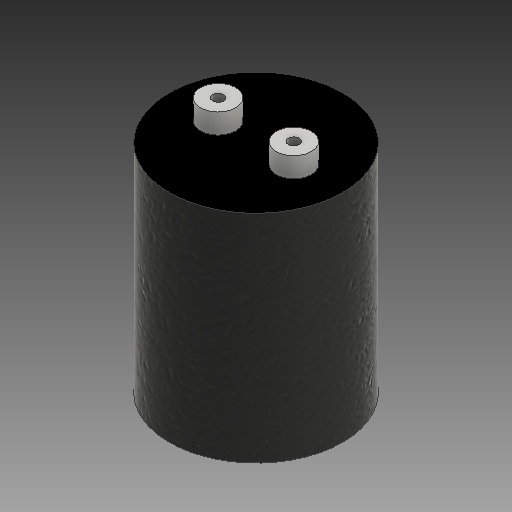
# Autodesk Inventor part: Capw
Saved by Autodesk Inventor 2019 (Build 230136000, 136)
## iProperties
Created: 2018-04-27
Part Number: Capw
Material: Generic
Document SubType Name: Modeling
Designer: Phil Erle
Density: 1 g/cm^3
Appearance: Aluminum - Dark
Author: Phil Erle
Autodesk Inventor part; units mm, degrees
ref_plane "YZ Plane" through (0, 0, 0) normal (1, 0, 0) x (0, 1, 0)
ref_plane "XZ Plane" through (0, 0, 0) normal (0, 1, 0) x (-1, 0, 0)
ref_plane "XY Plane" through (0, 0, 0) normal (0, 0, 1) x (1, 0, 0)
sketch "Sketch1" plane through (0, 0, 0) normal (0, 0, 1) x (1, 0, 0)
  circle A0 centre (0, 0) radius 32
  dimension "d0" = 64
  constraints: 1 centre point, 1 coincident
  measures "d0" diameter of A0
extrude "Extrusion1" add sketch "Sketch1" along normal blind 80
sketch "Sketch2" plane through (0, 0, 80) normal (0, 0, 1) x (1, 0, 0)
  line L0 (-14, 0) -> (14, 0) construction
  circle A0 centre (14, 0) radius 6.5
  circle A1 centre (-14, 0) radius 6.5
  point P0 (0, 0)
  point P1 (0, 0)
  dimension "d3" = 28
  dimension "d4" = 13
  dimension "d5" = 13
  constraints: 3 coincident, 2 centre point, 2 end point, 1 horizontal, 1 horizontal alignment, 1 midpoint
  measures "d3" distance of L0.start L0.end
  measures "d4" diameter of A0
  measures "d5" diameter of A1
extrude "Extrusion2" add sketch "Sketch2" along normal blind 7.4
sketch "Sketch3" plane through (-14, 0, 87.4) normal (0, 0, 1) x (1, 0, 0)
  point P0 (14, 0)
  point P1 (0, 0)
  point P2 (28, 0)
  dimension "d8" = 28
  dimension "d9" = 14
  constraints: 2 horizontal alignment
  measures "d8" distance of point (28, 0) point (0, 0)
  measures "d9" distance of point (14, 0) point (28, 0)
hole "Hole1" at (-14, 0, 87.4) at (14, 0, 87.4) direction (0, 0, -1) diameter 4.134 depth 14.2 tip angle 118 thread size "M5x0.8" class "6H" standard "ISO Metric profile"
body "Solid1"
